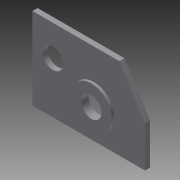
# Autodesk Inventor part: HW 2 Part 2
Saved by Autodesk Inventor 2015 SP1 (Build 190203100, 203)
## iProperties
Created: 2016-01-20
Part Number: HW 2 Part 2
Material: Generic
Document SubType Name: Modeling
Designer: melissa.roth
Density: 1 g/cm^3
Appearance: Default
Author: melissa.roth
Autodesk Inventor part; units mm, degrees
ref_plane "YZ Plane" through (0, 0, 0) normal (1, 0, 0) x (0, 1, 0)
ref_plane "XZ Plane" through (0, 0, 0) normal (0, 1, 0) x (-1, 0, 0)
ref_plane "XY Plane" through (0, 0, 0) normal (0, 0, 1) x (1, 0, 0)
sketch "Sketch1" plane through (0, 0, 0) normal (0, 0, 1) x (1, 0, 0)
  line L0 (0, 0) -> (0, 101.6)
  line L1 (0, 101.6) -> (107.95, 101.6)
  line L2 (107.95, 101.6) -> (139.7, 50.8)
  line L3 (139.7, 50.8) -> (139.7, 0)
  line L4 (139.7, 0) -> (0, 0)
  circle A0 centre (25.4, 63.5) radius 12.7
  circle A1 centre (76.2, 38.1) radius 25.4
  circle A2 centre (76.2, 38.1) radius 12.7
  dimension "d0" = 101.6
  dimension "d1" = 139.7
  dimension "d2" = 107.95
  dimension "d3" = 50.8
  dimension "d4" = 25.4
  dimension "d5" = 63.5
  dimension "d6" = 25.4
  dimension "d7" = 50.8
  dimension "d8" = 76.2
  dimension "d9" = 38.1
  dimension "d10" = 25.4
  constraints: 10 end point, 3 centre point, 2 perpendicular, 1 coincident, 1 parallel, 1 vertical
  measures "d0" distance of L0.start L0.end
  measures "d1" distance of L3.end L0.start
  measures "d2" distance of L0.end L1.end
  measures "d3" distance of L2.end L3.end
  measures "d4" diameter of A0
  measures "d5" distance from line of L4 A0.centre
  measures "d6" distance from line of L0 A0.centre
  measures "d7" diameter of A1
  measures "d8" distance from line of L0 A1.centre
  measures "d9" distance from line of L4 A1.centre
  measures "d10" diameter of A2
extrude "Extrusion1" add sketch "Sketch1" along normal blind 6.35 contours L0 L1 L2 L3 L4 | A1
sketch "Sketch2" plane through (0, 0, 6.35) normal (0, 0, 1) x (1, 0, 0)
  circle A0 centre (76.2, 38.1) radius 25.4
  line L0 (0, 101.6) -> (0, 0) projected
  line L1 (0, 0) -> (139.7, 0) projected
  circle A1 centre (76.2, 38.1) radius 12.7
  dimension "d13" = 50.8
  dimension "d14" = 76.2
  dimension "d15" = 38.1
  dimension "d16" = 25.4
  constraints: 2 centre point, 1 coincident
  measures "d13" diameter of A0
  measures "d14" distance from line of L0 A0.centre
  measures "d15" distance from line of L1 A0.centre
  measures "d16" diameter of A1
extrude "Extrusion2" add sketch "Sketch2" along normal blind 3.175
body "Solid1"
